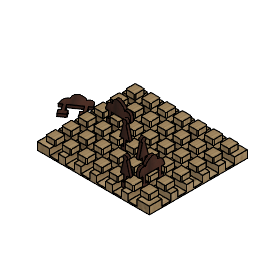
modelojoao (Autodesk Fusion 360 design; units mm, degrees)
Autodesk Fusion 360 part; units mm, degrees
sketch "Sketch1" plane through (0, 0, 0) normal (0, 0, 1) x (1, 0, 0) in component "Base"
  line L0 (0, 0) -> (400, 0)
  line L1 (400, 0) -> (400, 350)
  line L2 (400, 350) -> (0, 350)
  line L3 (0, 350) -> (0, 0)
  dimension "d6" = 400
  dimension "d7" = 350
  constraint horizontal L0
  constraint vertical L1
  constraint horizontal L2
  constraint vertical L3
  constraint coincident L0.start L3.end
  measures "d6" distance of L0.start L0.end
  measures "d7" distance of L0.start L2.end
extrude "Extrude1" add sketch "Sketch1" along normal blind 27 makes body 1 in component "Base"
sketch "Sketch1 (2)" plane through (0, 0, 0) normal (0, -1, 0) x (1, 0, 0) in component "Base"
  line L0 (0, 0) -> (400, 0)
  line L1 (400, 0) -> (400, 27)
  line L2 (400, 27) -> (0, 27)
  line L3 (0, 27) -> (0, 0)
  line L4 (0, 27) -> (20, 27)
  line L5 (20, 27) -> (44, 27)
  line L6 (44, 27) -> (76, 27)
  line L7 (76, 27) -> (100, 27)
  line L8 (100, 27) -> (132, 27)
  line L9 (132, 27) -> (156, 27)
  line L10 (156, 27) -> (188, 27)
  line L11 (188, 27) -> (212, 27)
  line L12 (212, 27) -> (244, 27)
  line L13 (244, 27) -> (268, 27)
  line L14 (268, 27) -> (300, 27)
  line L15 (300, 27) -> (324, 27)
  line L16 (324, 27) -> (356, 27)
  line L17 (356, 27) -> (380, 27)
  line L18 (380, 27) -> (400, 27)
  line L19 (44, 27) -> (76, 27)
  line L20 (76, 27) -> (76, 5)
  line L21 (76, 5) -> (44, 5)
  line L22 (44, 5) -> (44, 27)
  line L23 (100, 27) -> (132, 27)
  line L24 (132, 27) -> (132, 5)
  line L25 (132, 5) -> (100, 5)
  line L26 (100, 5) -> (100, 27)
  line L27 (156, 27) -> (188, 27)
  line L28 (188, 27) -> (188, 5)
  line L29 (188, 5) -> (156, 5)
  line L30 (156, 5) -> (156, 27)
  line L31 (212, 27) -> (244, 27)
  line L32 (244, 27) -> (244, 5)
  line L33 (244, 5) -> (212, 5)
  line L34 (212, 5) -> (212, 27)
  line L35 (268, 27) -> (300, 27)
  line L36 (300, 27) -> (300, 5)
  line L37 (300, 5) -> (268, 5)
  line L38 (268, 5) -> (268, 27)
  line L39 (324, 27) -> (356, 27)
  line L40 (356, 27) -> (356, 5)
  line L41 (356, 5) -> (324, 5)
  line L42 (324, 5) -> (324, 27)
  dimension "d10" = 20
  dimension "d11" = 24
  dimension "d12" = 32
  dimension "d13" = 24
  dimension "d14" = 32
  dimension "d15" = 24
  dimension "d16" = 32
  dimension "d17" = 24
  dimension "d18" = 32
  dimension "d19" = 24
  dimension "d20" = 32
  dimension "d21" = 24
  dimension "d22" = 32
  dimension "d23" = 24
  dimension "d24" = 20
  dimension "d26" = 32
  dimension "d27" = 22
  dimension "d28" = 32
  dimension "d29" = 22
  dimension "d30" = 32
  dimension "d31" = 22
  dimension "d32" = 32
  dimension "d33" = 22
  dimension "d34" = 32
  dimension "d35" = 22
  dimension "d36" = 32
  dimension "d37" = 22
  constraint coincident L2.end L3.start
  constraint perpendicular L3 L4
  constraint parallel L2 L5
  constraint parallel L2 L6
  constraint parallel L2 L7
  constraint parallel L2 L8
  constraint parallel L2 L9
  constraint parallel L2 L10
  constraint parallel L2 L11
  constraint coincident L2 L12.end
  constraint parallel L2 L13
  constraint parallel L2 L14
  constraint parallel L2 L15
  constraint parallel L15 L16
  constraint parallel L16 L17
  constraint parallel L17 L18
  constraint horizontal L19
  constraint vertical L20
  constraint horizontal L21
  constraint vertical L22
  constraint horizontal L23
  constraint vertical L24
  constraint horizontal L25
  constraint vertical L26
  constraint horizontal L27
  constraint vertical L28
  constraint horizontal L29
  constraint vertical L30
  constraint horizontal L31
  constraint vertical L32
  constraint horizontal L33
  constraint vertical L34
  constraint horizontal L35
  constraint vertical L36
  constraint horizontal L37
  constraint vertical L38
  constraint horizontal L39
  constraint vertical L40
  constraint horizontal L41
  constraint vertical L42
  measures "d10" distance of L2.end L4.end
  measures "d11" distance of L4.end L5.end
  measures "d12" distance of L5.end L6.end
  measures "d13" distance of L6.end L7.end
  measures "d14" distance of L7.end L8.end
  measures "d15" distance of L8.end L9.end
  measures "d16" distance of L9.end L10.end
  measures "d17" distance of L10.end L11.end
  measures "d18" distance of L11.end L12.end
  measures "d19" distance of L12.end L13.end
  measures "d20" distance of L13.end L14.end
  measures "d21" distance of L14.end L15.end
  measures "d22" distance of L15.end L16.end
  measures "d23" distance of L16.end L17.end
  measures "d24" distance of L17.end L1.end
  measures "d26" distance of L5.end L6.end
  measures "d27" distance of L5.end L21.end
  measures "d28" distance of L7.end L8.end
  measures "d29" distance of L7.end L25.end
  measures "d30" distance of L9.end L10.end
  measures "d31" distance of L9.end L29.end
  measures "d32" distance of L11.end L12.end
  measures "d33" distance of L11.end L33.end
  measures "d34" distance of L13.end L14.end
  measures "d35" distance of L13.end L37.end
  measures "d36" distance of L15.end L16.end
  measures "d37" distance of L15.end L41.end
extrude "Extrude2" cut sketch "Sketch1 (2)" against normal blind 350 contours L2 L6 L19 L20 L21 L22 | L2 L16 L39 L40 L41 L42 | L2 L8 L23 L24 L25 L26 | L2 L14 L35 L36 L37 L38 | L2 L10 L27 L28 L29 L30 | L2 L12 L31 L32 L33 L34 bodies 1 in component "Base"
sketch "Sketch2" plane through (0, 0, 0) normal (-1, 0, 0) x (0, -1, 0) in component "Base"
  line L0 (-350, 0) -> (0, 0)
  line L1 (0, 0) -> (0, 27)
  line L2 (0, 27) -> (-350, 27)
  line L3 (-350, 27) -> (-350, 0)
  line L4 (-350, 27) -> (-330, 27)
  line L5 (-330, 27) -> (-305, 27)
  line L6 (-305, 27) -> (-273, 27)
  line L7 (-273, 27) -> (-248, 27)
  line L8 (-248, 27) -> (-216, 27)
  line L9 (-216, 27) -> (-191, 27)
  line L10 (-191, 27) -> (-159, 27)
  line L11 (-159, 27) -> (-134, 27)
  line L12 (-134, 27) -> (-102, 27)
  line L13 (-102, 27) -> (-77, 27)
  line L14 (-77, 27) -> (-45, 27)
  line L15 (-45, 27) -> (-20, 27)
  line L16 (-20, 27) -> (0, 27)
  line L17 (-305, 27) -> (-273, 27)
  line L18 (-273, 27) -> (-273, 5)
  line L19 (-273, 5) -> (-305, 5)
  line L20 (-305, 5) -> (-305, 27)
  line L21 (-248, 27) -> (-216, 27)
  line L22 (-216, 27) -> (-216, 5)
  line L23 (-216, 5) -> (-248, 5)
  line L24 (-248, 5) -> (-248, 27)
  line L25 (-191, 27) -> (-159, 27)
  line L26 (-159, 27) -> (-159, 5)
  line L27 (-159, 5) -> (-191, 5)
  line L28 (-191, 5) -> (-191, 27)
  line L29 (-134, 27) -> (-102, 27)
  line L30 (-102, 27) -> (-102, 5)
  line L31 (-102, 5) -> (-134, 5)
  line L32 (-134, 5) -> (-134, 27)
  line L33 (-77, 27) -> (-45, 27)
  line L34 (-45, 27) -> (-45, 5)
  line L35 (-45, 5) -> (-77, 5)
  line L36 (-77, 5) -> (-77, 27)
  dimension "d40" = 20
  dimension "d41" = 25
  dimension "d42" = 32
  dimension "d43" = 25
  dimension "d44" = 32
  dimension "d45" = 25
  dimension "d46" = 32
  dimension "d47" = 25
  dimension "d48" = 32
  dimension "d49" = 25
  dimension "d50" = 32
  dimension "d51" = 25
  dimension "d52" = 20
  dimension "d53" = 32
  dimension "d54" = 22
  dimension "d55" = 32
  dimension "d56" = 22
  dimension "d57" = 32
  dimension "d58" = 22
  dimension "d59" = 32
  dimension "d60" = 22
  dimension "d61" = 32
  dimension "d62" = 22
  constraint coincident L2.end L3.start
  constraint perpendicular L3 L4
  constraint parallel L2 L5
  constraint parallel L2 L6
  constraint parallel L2 L7
  constraint parallel L2 L8
  constraint parallel L2 L9
  constraint parallel L2 L10
  constraint parallel L2 L11
  constraint parallel L2 L12
  constraint parallel L2 L13
  constraint parallel L2 L14
  constraint parallel L2 L15
  constraint perpendicular L1 L16
  constraint horizontal L17
  constraint vertical L18
  constraint horizontal L19
  constraint vertical L20
  constraint horizontal L21
  constraint vertical L22
  constraint horizontal L23
  constraint vertical L24
  constraint horizontal L25
  constraint vertical L26
  constraint horizontal L27
  constraint vertical L28
  constraint horizontal L29
  constraint vertical L30
  constraint horizontal L31
  constraint vertical L32
  constraint horizontal L33
  constraint vertical L34
  constraint horizontal L35
  constraint vertical L36
  measures "d40" distance of L2.end L4.end
  measures "d41" distance of L4.end L5.end
  measures "d42" distance of L5.end L6.end
  measures "d43" distance of L6.end L7.end
  measures "d44" distance of L7.end L8.end
  measures "d45" distance of L8.end L9.end
  measures "d46" distance of L9.end L10.end
  measures "d47" distance of L10.end L11.end
  measures "d48" distance of L11.end L12.end
  measures "d49" distance of L12.end L13.end
  measures "d50" distance of L13.end L14.end
  measures "d51" distance of L14.end L15.end
  measures "d52" distance of L15.end L1.end
  measures "d53" distance of L5.end L6.end
  measures "d54" distance of L5.end L19.end
  measures "d55" distance of L7.end L8.end
  measures "d56" distance of L7.end L23.end
  measures "d57" distance of L9.end L10.end
  measures "d58" distance of L9.end L27.end
  measures "d59" distance of L11.end L12.end
  measures "d60" distance of L11.end L31.end
  measures "d61" distance of L13.end L14.end
  measures "d62" distance of L13.end L35.end
extrude "Extrude3" cut sketch "Sketch2" against normal blind 400 contours L2 L6 L17 L18 L19 L20 | L2 L14 L33 L34 L35 L36 | L2 L8 L21 L22 L23 L24 | L2 L12 L29 L30 L31 L32 | L2 L10 L25 L26 L27 L28 bodies 1 in component "Base"
sketch "Sketch3" plane through (0, 0, 27) normal (0, 0, 1) x (-1, 0, 0) in component "Base"
  line L0 (-44, -45) -> (0, -45)
  line L1 (0, -45) -> (0, 0)
  line L2 (0, 0) -> (-44, 0)
  line L3 (-44, 0) -> (-44, -45)
  line L4 (-44, 0) -> (-44, -20)
  line L5 (0, -45) -> (-20, -45)
  line L6 (-20, -45) -> (-44, -45)
  line L7 (-44, -45) -> (-44, -20)
  line L8 (-44, -20) -> (-20, -20)
  line L9 (-20, -20) -> (-20, -45)
  line L10 (-20, -45) -> (-44, -20) construction
  circle A0 centre (-32, -32.5) radius 5
  dimension "d65" = 20
  dimension "d66" = 20
  dimension "d67" = 10
  constraint coincident L2.end L3.start
  constraint perpendicular L2 L4
  constraint coincident L0.end L1.start
  constraint perpendicular L1 L5
  constraint horizontal L6
  constraint vertical L7
  constraint horizontal L8
  constraint vertical L9
  constraint midpoint L10 A0.centre
  measures "d65" distance of L2.end L4.end
  measures "d66" distance of L0.end L5.end
  measures "d67" diameter of A0
extrude "Extrude4" add sketch "Sketch3" along normal blind 10 contours A0 bodies 1 in component "Base"
pattern_linear "R-Pattern1" count 7 spacing 56 along (1, 0, 0) count 6 spacing 57 along (0, 1, 0) of "Extrude4" in component "Base"
sketch "Sketch1 (3)" plane through (0, 0, 37) normal (0, 0, 1) x (-1, 0, 0) in component "Tampas"
  circle A0 centre (-32, -32.5) radius 5
  line L0 (-15, -15) -> (-49, -15)
  line L1 (-49, -15) -> (-49, -50)
  line L2 (-49, -50) -> (-15, -50)
  line L3 (-15, -50) -> (-15, -15)
  line L4 (-15, -15) -> (-49, -50) construction
  line L5 (-49, -15) -> (-15, -50) construction
  circle A1 centre (-32, -32.5) radius 6.5
  point P0 (-32, -32.5)
  dimension "d74" = 34
  dimension "d75" = 35
  dimension "d82" = 13
  constraint horizontal L0
  constraint perpendicular L0 L1
  constraint parallel L0 L2
  constraint parallel L1 L3
  constraint coincident L4 P0
  constraint coincident L5 P0
  constraint coincident P0 A0.centre
  constraint concentric A0 A1
  measures "d74" distance of L1.end L2.end
  measures "d75" distance of L0.end L1.end
  measures "d82" diameter of A1
extrude "Extrude1'" add sketch "Sketch1 (3)" along normal blind 18 separate body contours A0 | L0 L1 L2 L3 | A1 makes body 2 in component "Tampas"
extrude "Extrude3'" cut sketch "Sketch1 (3)" along normal blind 10 contours A0 | A1 bodies 2 in component "Tampas"
fillet "Fillet2" radius 3 4 edges at (15, 15, 46) (49, 15, 46) (15, 50, 46) (49, 50, 46) on bodies 2 in component "Tampas"
pattern_linear "R-Pattern1'" count 7 spacing 56 along (1, 0, 0) count 6 spacing 57 along (0, 1, 0) of bodies 2 makes body 3 at (82.3333, 37.3333, 55) makes body 4 at (138.3333, 37.3333, 55) makes body 5 at (194.3333, 37.3333, 55) makes body 6 at (250.3333, 37.3333, 55) makes body 7 at (306.3333, 37.3333, 55) makes body 8 at (362.3333, 37.3333, 55) makes body 9 at (37.6667, 94.3333, 55) makes body 10 at (82.3333, 94.3333, 55) makes body 11 at (138.3333, 94.3333, 55) makes body 12 at (194.3333, 94.3333, 55) makes body 13 at (250.3333, 94.3333, 55) makes body 14 at (317.6667, 84.6667, 55) makes body 15 at (373.6667, 84.6667, 55) makes body 16 at (37.6667, 151.3333, 55) makes body 17 at (82.3333, 151.3333, 55) makes body 18 at (138.3333, 151.3333, 55) makes body 19 at (194.3333, 151.3333, 55) makes body 20 at (250.3333, 151.3333, 55) makes body 21 at (317.6667, 141.6667, 55) makes body 22 at (373.6667, 141.6667, 55) makes body 23 at (37.6667, 208.3333, 55) makes body 24 at (82.3333, 208.3333, 55) makes body 25 at (138.3333, 208.3333, 55) makes body 26 at (194.3333, 208.3333, 55) makes body 27 at (250.3333, 208.3333, 55) makes body 28 at (317.6667, 198.6667, 55) makes body 29 at (373.6667, 198.6667, 55) makes body 30 at (26.3333, 265.3333, 55) makes body 31 at (82.3333, 265.3333, 55) makes body 32 at (138.3333, 265.3333, 55) makes body 33 at (194.3333, 265.3333, 55) makes body 34 at (250.3333, 265.3333, 55) makes body 35 at (306.3333, 265.3333, 55) makes body 36 at (362.3333, 265.3333, 55) makes body 37 at (26.3333, 322.3333, 55) makes body 38 at (82.3333, 322.3333, 55) makes body 39 at (138.3333, 322.3333, 55) makes body 40 at (194.3333, 322.3333, 55) makes body 41 at (250.3333, 322.3333, 55) makes body 42 at (306.3333, 322.3333, 55) makes body 43 at (362.3333, 322.3333, 55) in component "Tampas"
sketch "Sketch1 (4)" plane through (0, 0, 0) normal (0, -1, 0) x (1, 0, 0) in component "boneco1"
  line L0 (212, 5) -> (212, 27)
  line L1 (212, 27) -> (188, 27)
  line L2 (188, 27) -> (188, 5)
  line L3 (188, 5) -> (156, 5)
  line L4 (156, 5) -> (156, 27)
  line L5 (156, 27) -> (132, 27)
  line L6 (132, 27) -> (132, 5)
  line L7 (132, 5) -> (100, 5)
  line L8 (100, 5) -> (100, 27)
  line L9 (100, 27) -> (76, 27)
  line L10 (76, 27) -> (76, 5)
  line L11 (76, 5) -> (44, 5)
  line L12 (44, 5) -> (44, 27)
  line L13 (44, 27) -> (0, 27)
  line L14 (0, 27) -> (0, 0)
  line L15 (0, 0) -> (400, 0)
  line L16 (400, 0) -> (400, 27)
  line L17 (400, 27) -> (356, 27)
  line L18 (356, 27) -> (356, 5)
  line L19 (356, 5) -> (324, 5)
  line L20 (324, 5) -> (324, 27)
  line L21 (324, 27) -> (300, 27)
  line L22 (300, 27) -> (300, 5)
  line L23 (300, 5) -> (268, 5)
  line L24 (268, 5) -> (268, 27)
  line L25 (268, 27) -> (244, 27)
  line L26 (244, 27) -> (244, 5)
  line L27 (244, 5) -> (212, 5)
  line L28 (44, 27) -> (47, 27)
  line L29 (47, 27) -> (47, 26)
  line L30 (47, 26) -> (73, 26)
  line L31 (73, 26) -> (73, 8)
  line L32 (73, 8) -> (47, 8)
  line L33 (47, 8) -> (47, 26)
  line L34 (55, 26) -> (65, 26)
  line L35 (65, 26) -> (65, 50)
  line L36 (65, 50) -> (55, 50)
  line L37 (55, 50) -> (55, 26)
  line L38 (55, 50) -> (43, 50)
  line L39 (65, 50) -> (77, 50)
  line L40 (60, 50) -> (60, 100)
  line L41 (60, 100) -> (64, 100)
  line L42 (60, 100) -> (56, 100)
  line L43 (64, 100) -> (77, 50)
  line L44 (56, 100) -> (43, 50)
  circle A0 centre (60, 104) radius 8
  constraint coincident L12.end L13.start
  constraint perpendicular L12 L28
  constraint perpendicular L28 L29
  constraint horizontal L30
  constraint vertical L31
  constraint horizontal L32
  constraint vertical L33
  constraint horizontal L34
  constraint vertical L35
  constraint horizontal L36
  constraint vertical L37
  constraint coincident L30 L34.start
  constraint perpendicular L37 L38
  constraint perpendicular L35 L39
  constraint midpoint L36 L40.start
  constraint perpendicular L36 L40
  constraint perpendicular L40 L41
  constraint perpendicular L40 L42
extrude "Extrude1''" add sketch "Sketch1 (4)" along normal blind 10 separate body contours L30 L31 L32 L33 L34 | L30 L34 L35 L36 L37 | L36 L38 L40 L44 A0 | L36 L39 L40 L43 A0 | L40 L42 L44 A0 | L40 L41 L43 A0 | L41 L42 L43 L44 A0 makes body 44 in component "boneco1"
move_body "Move1" bodies 44 to x (1, 0, 0) y (0, 1, 0) z (0, 0, 1) at (112, 150, 0) in component "boneco1"
copy_body "CopyPasteBodies1" bodies 44 makes body 45 in component "boneco1"
move_body "Move2" bodies 45 to x (1, 0, 0) y (0, 1, 0) z (0, 0, 1) at (112, -110, 0) in component "boneco1"
copy_body "CopyPasteBodies2" bodies 44 makes body 46 in component "boneco1"
move_body "Move3" bodies 46 to x (0, -1, 0) y (1, 0, 0) z (0, 0, 1) at (112, 290, 0) in component "boneco1"
sketch "Sketch1 (5)" plane through (0, 0, 0) normal (0, -1, 0) x (1, 0, 0) in component "Cenário"
  line L0 (212, 5) -> (212, 27)
  line L1 (212, 27) -> (188, 27)
  line L2 (188, 27) -> (188, 5)
  line L3 (188, 5) -> (156, 5)
  line L4 (156, 5) -> (156, 27)
  line L5 (156, 27) -> (132, 27)
  line L6 (132, 27) -> (132, 5)
  line L7 (132, 5) -> (100, 5)
  line L8 (100, 5) -> (100, 27)
  line L9 (100, 27) -> (76, 27)
  line L10 (76, 27) -> (76, 5)
  line L11 (76, 5) -> (44, 5)
  line L12 (44, 5) -> (44, 27)
  line L13 (44, 27) -> (0, 27)
  line L14 (0, 27) -> (0, 0)
  line L15 (0, 0) -> (400, 0)
  line L16 (400, 0) -> (400, 27)
  line L17 (400, 27) -> (356, 27)
  line L18 (356, 27) -> (356, 5)
  line L19 (356, 5) -> (324, 5)
  line L20 (324, 5) -> (324, 27)
  line L21 (324, 27) -> (300, 27)
  line L22 (300, 27) -> (300, 5)
  line L23 (300, 5) -> (268, 5)
  line L24 (268, 5) -> (268, 27)
  line L25 (268, 27) -> (244, 27)
  line L26 (244, 27) -> (244, 5)
  line L27 (244, 5) -> (212, 5)
  line L28 (47, 26) -> (73, 26)
  line L29 (73, 26) -> (73, 8)
  line L30 (73, 8) -> (47, 8)
  line L31 (47, 8) -> (47, 26)
  line L32 (55, 26) -> (65, 26)
  line L33 (65, 26) -> (65, 50)
  line L34 (65, 50) -> (55, 50)
  line L35 (55, 50) -> (55, 26)
  line L36 (121, 26) -> (121, 50)
  line L37 (121, 50) -> (111, 50)
  line L38 (111, 50) -> (111, 26)
  line L39 (103, 8) -> (103, 26)
  line L40 (129, 8) -> (103, 8)
  line L41 (129, 26) -> (129, 8)
  line L42 (103, 26) -> (129, 26)
  line L43 (55, 50) -> (43, 50)
  line L44 (65, 50) -> (111, 50)
  line L45 (121, 50) -> (133, 50)
  spline S0 degree 5 poles (43, 50) (43.2725, 51.1469) (43.8367, 53.3946) (44.741, 56.6278) (46.0645, 60.6574) (47.9295, 65.1912) (50.0276, 69.1682) (52.3844, 72.527) (55.0231, 75.2125) (57.9512, 77.2065) (61.1556, 78.5408) (63.9258, 79.1142) (66.113, 79.2825) (67.6191, 79.2803) (68.3841, 79.2505) knots 0 0 0 0 0 0 0.1 0.2 0.3 0.4 0.5 0.6 0.7 0.8 0.9 1 1 1 1 1 1
  spline S1 degree 5 poles (68.3841, 79.2505) (68.5028, 79.9689) (68.7657, 81.3749) (69.236, 83.3916) (70.0157, 85.8955) (71.2447, 88.7129) (72.7241, 91.2112) (74.4424, 93.3807) (76.378, 95.2086) (78.495, 96.6793) (80.7404, 97.7746) (83.0549, 98.4784) (85.3827, 98.7823) (87.6807, 98.6897) (89.9305, 98.2224) (92.1415, 97.4224) (94.3352, 96.3428) (96.5324, 95.0411) (98.7405, 93.5718) (100.9376, 91.979) (103.0709, 90.2927) (105.0706, 88.5336) (106.861, 86.7141) (108.3715, 84.8413) (109.549, 82.9192) (110.3655, 80.9505) (110.7203, 79.3398) (110.8177, 78.1118) (110.8078, 77.2844) (110.7842, 76.8685) knots 0 0 0 0 0 0 0.04 0.08 0.12 0.16 0.2 0.24 0.28 0.32 0.36 0.4 0.44 0.48 0.52 0.56 0.6 0.64 0.68 0.72 0.76 0.8 0.84 0.88 0.92 0.96 1 1 1 1 1 1
  spline S2 degree 5 poles (110.7842, 76.8685) (111.127, 77.0528) (111.8299, 77.4065) (112.9366, 77.8929) (114.5179, 78.4522) (116.666, 78.99) (118.9649, 79.3352) (121.365, 79.4302) (123.7783, 79.1842) (126.0977, 78.4919) (128.2144, 77.2503) (130.035, 75.3758) (131.5025, 72.8276) (132.5891, 69.597) (133.286, 65.6942) (133.5965, 61.139) (133.5423, 56.9901) (133.3354, 53.6018) (133.124, 51.2209) (133, 50) knots 0 0 0 0 0 0 0.066667 0.133333 0.2 0.266667 0.333333 0.4 0.466667 0.533333 0.6 0.666667 0.733333 0.8 0.866667 0.933333 1 1 1 1 1 1
  point P0 (54.2111, 74.2483)
  point P1 (76.2448, 94.9719)
  point P2 (86.9639, 98.6641)
  point P3 (97.6831, 94.2573)
  point P4 (107.9258, 85.3247)
  point P5 (118.764, 79.2505)
  point P6 (128.4112, 76.8685)
  dimension "d93" = 12
  dimension "d94" = 12
  constraint horizontal L28
  constraint vertical L29
  constraint horizontal L30
  constraint vertical L31
  constraint horizontal L32
  constraint vertical L33
  constraint horizontal L34
  constraint vertical L35
  constraint coincident L28 L32.start
  constraint horizontal L42
  constraint vertical L41
  constraint horizontal L40
  constraint vertical L39
  constraint vertical L36
  constraint horizontal L37
  constraint vertical L38
  constraint coincident L38.end L42
  constraint perpendicular L35 L43
  constraint perpendicular L38 L44
  constraint perpendicular L36 L45
  measures "d93" distance of L34.end L43.end
  measures "d94" distance of L36.end L45.end
extrude "Extrude1'''" add sketch "Sketch1 (5)" along normal blind 10 separate body contours L28 L29 L30 L31 L32 | L28 L32 L33 L34 L35 | L34 L37 L43 L44 L45 S0 S1 S2 | L36 L37 L38 L42 | L39 L40 L41 L42 makes body 47 in component "Cenário"
move_body "Move1'" bodies 47 to x (1, 0, 0) y (0, 1, 0) z (0, 0, 1) at (0, 210, 0) in component "Cenário"
copy_body "CopyPasteBodies1'" bodies 47 makes body 48 in component "Cenário"
move_body "Move2'" bodies 48 to x (0, -1, 0) y (1, 0, 0) z (0, 0, 1) at (110.2347, 178.2347, 0) in component "Cenário"
copy_body "CopyPasteBodies2'" bodies 47 makes body 49 in component "Cenário"
move_body "Move3'" bodies 49 to x (0.819152, 0.573576, 0) y (0, 0, -1) z (-0.573576, 0.819152, 0) at (-103.4352, 105.6684, 210.3532) in component "Cenário"
component "Base" placed x (1, 0, 0) y (0, 1, 0) z (0, 0, 1) at (0, 0, 0)
component "Tampas" placed x (1, 0, 0) y (0, 1, 0) z (0, 0, 1) at (0, 0, -8)
component "boneco1" placed x (1, 0, 0) y (0, 1, 0) z (0, 0, 1) at (0, 0, 0)
component "Cenário" placed x (1, 0, 0) y (0, 1, 0) z (0, 0, 1) at (0, 0, 0)
equation "Xsize = 400 mm"
equation "Ysize = 350 mm"
equation "gap = 3 mm"
equation "gross1 = 27 mm"
equation "gross2 = 18 mm"
equation "d6 = Xsize"
equation "d7 = Ysize"
equation "d8 = gross1"
equation "d11 = ( ( Xsize - ( d10 * 2 ) ) - ( d12 * 6 ) ) / 7"
equation "d12 = 5 mm + gap * 2 + toy + gap * 2 + 5 mm"
equation "d13 = d11"
equation "d14 = d12"
equation "d15 = d11"
equation "d16 = d12"
equation "d17 = d11"
equation "d18 = d12"
equation "d19 = d11"
equation "d20 = d12"
equation "d21 = d11"
equation "d22 = d12"
equation "d23 = d11"
equation "toy = 10 mm"
equation "d26 = d12"
equation "d27 = gap * 4 + 10 mm"
equation "d28 = d12"
equation "d29 = d27"
equation "d30 = d12"
equation "d31 = d27"
equation "d32 = d12"
equation "d33 = d27"
equation "d34 = d12"
equation "d35 = d27"
equation "d36 = d12"
equation "d37 = d27"
equation "d38 = -Ysize"
equation "d40 = d10"
equation "d41 = ( ( Ysize - d10 * 2 ) - ( d12 * 5 ) ) / 6"
equation "d42 = d12"
equation "d43 = d41"
equation "d44 = d12"
equation "d45 = d41"
equation "d46 = d12"
equation "d47 = d41"
equation "d48 = d12"
equation "d49 = d41"
equation "d50 = d12"
equation "d51 = d41"
equation "d52 = d10"
equation "d53 = d12"
equation "d54 = d27"
equation "d55 = d12"
equation "d56 = d27"
equation "d57 = d12"
equation "d58 = d27"
equation "d59 = d12"
equation "d60 = d27"
equation "d61 = d12"
equation "d62 = d27"
equation "d63 = -Xsize"
equation "d65 = d10"
equation "d66 = d10"
equation "d74 = d11 + ( 5 * 2 ) * 1 mm"
equation "d75 = d41 + ( 5 * 2 ) * 1 mm"
equation "d76 = gross2"
equation "d82 = 10 mm + gap"
equation "d90 = gap"
